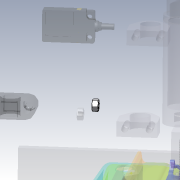
# Autodesk Inventor part: NUT, HEX, M4
Saved by Autodesk Inventor 2022.4 (Build 264492000, 492)
## iProperties
Manager: 100-14513
Category: _
Comments: To add or edit properties for Autodesk Inventor files, use iProperties.
Alert: To add or edit properties for Autodesk Inventor files, use iProperties.
Created: 2009-10-28
Part Number: NUT, HEX, M4
Vendor: Autodesk Inc.
Document SubType Name: Modeling
Designer: dan.vanderzwet
Material: Steel, MS
Description: NUT, HEX, M4
Standard: ANSI B18.2.4.2M
Checked By: 1VYKJ
Engr Approved By: R
User Status: Released
Mfg Approved By: -
Size Designation: M4 x 0.7
Density: 7.86 g/cm^3
Appearance: Rubber (Black)
Mass: 0.819831 g
Surface Area: 1.68005 cm^2
Volume: 0.104304 cm^3
Control State: 0
Master: False
Checked Out: False
Shininess: 64.0
Length Units: 11269
Angle Units: 11279
Time Units: 11290
Mass Units: 11283
Length Display Precision: 3
Angle Display Precision: 2
Compacted: True
CN_SERVICEABLE: _
FIRST_DESCRIPTION: NUT, HEX, M4
PTC_WM_ITERATION: 7
PTC_WM_ORGANIZATION_ID: CLWC
PTC_WM_LIFECYCLE: CLWC_CAD_LC
CN_MASS: 0.00082
SECOND_DESCRIPTION: _
THIRD_DESCRIPTION: _
CL_runCount: 1
FinishProperty: ToBeSet
CN_MFG_PART_NUM: _
Density: 0.0
Volumn: 0.0
Area: 0.0
PropertySet Name: Model Information
Title: NUT, HEX, M4_1VYKJ.ipt
Author: -
Keywords: -
Revision Number: 1
Subject: _
Autodesk Inventor part; units mm, degrees
ref_plane "YZ Plane" through (0, 0, 0) normal (1, 0, 0) x (0, 1, 0)
ref_plane "XZ Plane" through (0, 0, 0) normal (0, 1, 0) x (-1, 0, 0)
ref_plane "XY Plane" through (0, 0, 0) normal (0, 0, 1) x (1, 0, 0)
sketch "Sketch1" plane through (0, 0, 0) normal (1, 0, 0) x (0, 1, 0)
  line L0 (-4.0415, 0) -> (-2.0207, 3.5)
  line L1 (-2.0207, 3.5) -> (2.0207, 3.5)
  line L2 (2.0207, 3.5) -> (4.0415, 0)
  line L3 (4.0415, 0) -> (2.0207, -3.5)
  line L4 (2.0207, -3.5) -> (-2.0207, -3.5)
  line L5 (-2.0207, -3.5) -> (-4.0415, 0)
  point P0 (0, 0)
  point P1 (0, 0)
  dimension "d0" = 8.0829
  constraints: 12 end point, 1 coincident, 1 horizontal, 11 other
  measures "d0" distance of L2.end L0.start
extrude "Body" add sketch "Sketch1" along normal blind 3.1
sketch "Sketch2" plane through (0, 0, 0) normal (0, 0, 1) x (1, 0, 0)
  line L0 (0, 2.0207) -> (0, 4.0415) projected
  line L1 (0, 4.0415) -> (3.1, 4.0415) projected
  line L2 (3.1, 2.0207) -> (3.1, 4.0415) projected
  line L3 (-0.62, 0) -> (3.72, 0) projected
  line L4 (0.3126, 4.0415) -> (0, 3.5)
  line L5 (2.7874, 4.0415) -> (3.1, 3.5)
  dimension "d3" = 30
  dimension "d4" = 30
  dimension "d5" = 7
  dimension "d6" = 7
  constraints: 4 end point, 4 point on line
  measures "d3" angle of L0 L4
  measures "d4" angle of L2 L5
  measures "d5" diameter of L4.end L3
  measures "d6" diameter of L5.end L3
revolve "Chamfer1" cut sketch "Sketch2" angle 360 about axis through (-10, 0, 0) along (1, 0, 0)
sketch "Sketch3" plane through (3.1, 0, 0) normal (1, 0, 0) x (0, 0, -1)
  arc A0 (-1.75, -3.0311) -> (1.75, -3.0311) centre (0, 0) ccw projected
  constraints: 1 coincident
hole "Thread" at (3.1, 0, 0) direction (-1, 0, 0) diameter 3.242 end through all thread size "M4x0.7" class "6H" standard "ANSI Metric M Profile"
chamfer "Chamfer2" distance 0.3789 angle 30 1 edges at (3.1, 0, 1.621) measured on face at (3.1, 0, 2.121)
chamfer "Chamfer3" distance 0.3789 angle 30 1 edges at (0, 0, 1.621) measured on face at (0, 0, 2.121)
equation "\"d0\" = 1.1547 * SW"
equation "\"d3\" = ANG1"
equation "\"d4\" = ANG2"
equation "\"d5\" = SW0"
equation "\"d6\" = SW01"
equation "\"d8\" = -0.5 * GD1 + 0.5 * NND"
equation "\"d40\" = -0.5 * GD1 + 0.5 * NND"
equation "\"d10\" = -0.5 * GD1 + 0.5 * NND"
equation "\"d41\" = -0.5 * GD1 + 0.5 * NND"
equation "\"ANG1\" = 30deg"
equation "\"ANG2\" = 30deg"
equation "\"NND\" = 4"
equation "\"KOH\" = 3.8"
equation "\"SW\" = 7"
equation "\"SW0\" = SW"
equation "\"SW01\" = SW"
equation "\"E0\" = 1.155 * SW"
equation "\"THREADDIA\" = 4"
equation "\"TPU\" = 0.7"
equation "\"GUL\" = 0.541266 * TPU"
equation "\"GAL\" = 0.541266 * TPU"
equation "\"PTC\" = TPU"
equation "\"TOA\" = 30deg"
equation "\"GD1\" = 3.242228"
body "Solid1"
